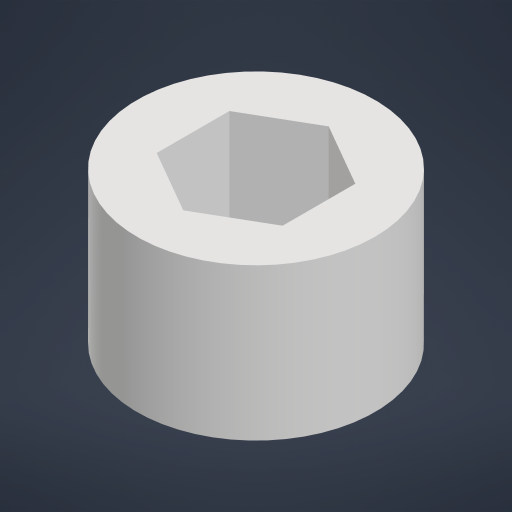
# Autodesk Inventor part: 5mm x 11.4mm Hex Spacer
Saved by Autodesk Inventor 2023 (Build 270158000, 158)
## iProperties
Created: 2022-10-05
Part Number: 5mm x 11.4mm Hex Spacer
Material: Generic
Document SubType Name: Modeling
Designer: izack
Density: 1 g/cm^3
Appearance: Default
Author: izack
## iProperties of the stored document 5mm x 9.9mm Hex Spacer_3DPrint.ipt
Part Number: 5mm x 9.9mm Hex Spacer_3DPrint
Material: Generic
Document SubType Name: Modeling
Designer: izack
Appearance: Default
Author: izack
Autodesk Inventor part; units mm, degrees
ref_plane "YZ Plane" through (0, 0, 0) normal (1, 0, 0) x (0, 1, 0)
ref_plane "XZ Plane" through (0, 0, 0) normal (0, 1, 0) x (-1, 0, 0)
ref_plane "Work Plane1" through (-28.2023, 6.3891, -28.2023) normal (0, -1, 0) x (0.9921, 0, 0.1251)
sketch "Sketch1" plane through (0, 0, 0) normal (0, 1, 0) x (-1, 0, 0)
  circle A0 centre (0, 0) radius 2.65
  line L0 (2.65, -1.53) -> (0, -3.06)
  line L1 (0, -3.06) -> (-2.65, -1.53)
  line L2 (-2.65, -1.53) -> (-2.65, 1.53)
  line L3 (-2.65, 1.53) -> (0, 3.06)
  line L4 (0, 3.06) -> (2.65, 1.53)
  line L5 (2.65, 1.53) -> (2.65, -1.53)
  circle A1 centre (0, 0) radius 5
  point P0 (2.65, 0)
  dimension "d0" = 5.3
  dimension "d1" = 10
  constraints: 12 end point, 3 coincident, 1 centre point, 1 horizontal alignment, 1 midpoint, 15 other
  measures "d1" diameter of A1
extrude "Extrusion1" add sketch "Sketch1" along normal up to surface (6.3891 mm away)
body "Solid1"
